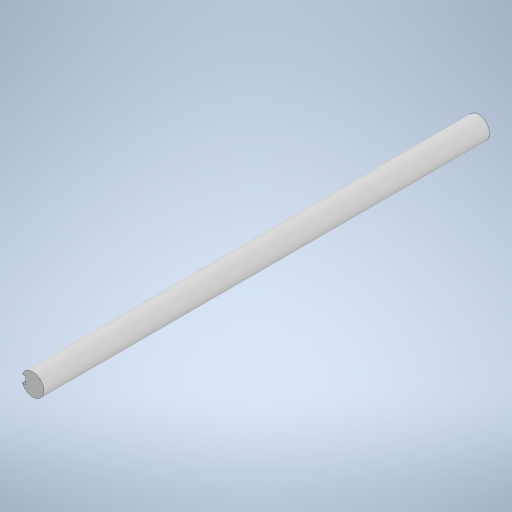
# Autodesk Inventor part: ShaftNutV1
Saved by Autodesk Inventor 2024.4 (Build 284460000, 460)
## iProperties
Created: 2025-11-05
Part Number: ShaftNutV1
Material: Generic
Document SubType Name: Modeling
Designer: jonas
Density: 1 g/cm^3
Appearance: Default
Author: jonas
Autodesk Inventor part; units mm, degrees
ref_plane "YZ Plane" through (0, 0, 0) normal (1, 0, 0) x (0, 1, 0)
ref_plane "XZ Plane" through (0, 0, 0) normal (0, 1, 0) x (-1, 0, 0)
ref_plane "XY Plane" through (0, 0, 0) normal (0, 0, 1) x (1, 0, 0)
sketch "Sketch1" plane through (0, 0, 0) normal (0, 1, 0) x (-1, 0, 0)
  line L0 (0, 10.4293) -> (0, -10.4293) construction
  line L1 (-2.2615, 0) -> (2.2615, 0) construction
  arc A0 (7.0711, 2.5) -> (7.0711, -2.5) centre (0, 0) ccw
  line L2 (7.0711, 2.5) -> (5, 2.5)
  line L3 (5, 2.5) -> (5, -2.5)
  line L4 (5, -2.5) -> (7.0711, -2.5)
  dimension "d0" = 15
  dimension "d1" = 5
  dimension "d2" = 5
  constraints: 10 end point, 2 coincident, 2 horizontal, 2 midpoint, 2 point on circle, 1 centre point, 1 parallel, 1 perpendicular, 1 vertical, 1 other
  measures "d0" diameter of A0
  measures "d1" distance of L2.end L3.end
  measures "d2" distance between parallel lines of L0 L3
extrude "Extrusion1" add sketch "Sketch1" along normal blind 300
body "Solid1"
